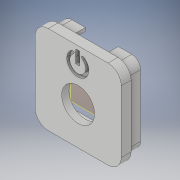
# Autodesk Inventor part: cap
Saved by Autodesk Inventor 2019 (Build 230136000, 136)
## iProperties
Created: 2019-08-20
Part Number: cap
Material: Generic
Document SubType Name: Modeling
Designer: assman
Density: 1 g/cm^3
Appearance: Default
Author: assman
## iProperties of the stored document cap_3DPrint.ipt
Created: 2019-08-20
Part Number: cap_3DPrint
Material: Generic
Document SubType Name: Modeling
Designer: assman
Density: 1 g/cm^3
Appearance: Default
Author: assman
Autodesk Inventor part; units mm, degrees
ref_plane "YZ Plane" through (0, 0, 0) normal (1, 0, 0) x (0, 1, 0)
ref_plane "XZ Plane" through (0, 0, 0) normal (0, 1, 0) x (-1, 0, 0)
ref_plane "XY Plane" through (0, 0, 0) normal (0, 0, 1) x (1, 0, 0)
ref_plane "Work Plane1" through (0, 0, 0) normal (0, 0, 1) x (1, 0, 0)
sketch "Sketch1" plane through (0, 0, 0) normal (0, 0, 1) x (1, 0, 0)
  line L0 (13.075, 9.425) -> (13.075, -9.425) projected
  arc A0 (13.075, 9.425) -> (9.075, 13.425) centre (9.075, 9.425) ccw projected
  line L1 (5, 13.425) -> (9.075, 13.425) projected
  line L2 (-4, 13.425) -> (4, 13.425) projected
  line L3 (5, 13.425) -> (4, 13.425) projected
  line L4 (-4, 13.425) -> (-5, 13.425) projected
  line L5 (-9.075, 13.425) -> (-5, 13.425) projected
  arc A1 (-9.075, 13.425) -> (-13.075, 9.425) centre (-9.075, 9.425) ccw projected
  line L6 (-13.075, -9.425) -> (-13.075, 9.425) projected
  arc A2 (-13.075, -9.425) -> (-9.075, -13.425) centre (-9.075, -9.425) ccw projected
  line L7 (9.075, -13.425) -> (-9.075, -13.425) projected
  arc A3 (9.075, -13.425) -> (13.075, -9.425) centre (9.075, -9.425) ccw projected
  point P0 (0, 0)
extrude "Extrusion1" add sketch "Sketch1" along normal blind 1.2
sketch "Sketch2" plane through (0, 0, 1.2) normal (0, 0, 1) x (1, 0, 0)
  circle A0 centre (0, -2) radius 3.85
  line L0 (-9.075, -13.425) -> (9.075, -13.425)
  point P0 (0, 0)
  dimension "d10" = 13.425
  dimension "d11" = 2
  constraints: 2 end point, 1 centre point
  measures "d10" distance from line of L0 point (0, 0)
  measures "d11" distance of point (0, 0) A0.centre
extrude "Extrusion2" cut sketch "Sketch2" against normal blind 1.2
sketch "Sketch3" plane through (0, 0, 0) normal (0, 0, -1) x (-1, 0, 0)
  arc A0 (-9.075, 12.225) -> (-11.875, 9.425) centre (-9.075, 9.425) ccw projected
  line L0 (-9.075, 12.225) -> (-5, 12.225) projected
  line L1 (-11.875, -9.425) -> (-11.875, 9.425) projected
  arc A1 (-11.875, -9.425) -> (-9.075, -12.225) centre (-9.075, -9.425) ccw projected
  line L2 (9.075, -12.225) -> (-9.075, -12.225) projected
  arc A2 (9.075, -12.225) -> (11.875, -9.425) centre (9.075, -9.425) ccw projected
  line L3 (11.875, 9.425) -> (11.875, -9.425) projected
  arc A3 (11.875, 9.425) -> (9.075, 12.225) centre (9.075, 9.425) ccw projected
  line L4 (5, 12.225) -> (9.075, 12.225) projected
  line L5 (5, 12.125) -> (9.075, 12.125)
  arc A4 (11.775, 9.425) -> (9.075, 12.125) centre (9.075, 9.425) ccw
  line L6 (11.775, 9.425) -> (11.775, -9.425)
  arc A5 (9.075, -12.125) -> (11.775, -9.425) centre (9.075, -9.425) ccw
  line L7 (9.075, -12.125) -> (-9.075, -12.125)
  arc A6 (-11.775, -9.425) -> (-9.075, -12.125) centre (-9.075, -9.425) ccw
  line L8 (-11.775, -9.425) -> (-11.775, 9.425)
  arc A7 (-9.075, 12.125) -> (-11.775, 9.425) centre (-9.075, 9.425) ccw
  line L9 (-9.075, 12.125) -> (-5, 12.125)
  line L10 (5, 11.125) -> (9.075, 11.125)
  arc A8 (10.775, 9.425) -> (9.075, 11.125) centre (9.075, 9.425) ccw
  line L11 (10.775, 9.425) -> (10.775, -9.425)
  arc A9 (9.075, -11.125) -> (10.775, -9.425) centre (9.075, -9.425) ccw
  line L12 (9.075, -11.125) -> (-9.075, -11.125)
  arc A10 (-10.775, -9.425) -> (-9.075, -11.125) centre (-9.075, -9.425) ccw
  line L13 (-10.775, -9.425) -> (-10.775, 9.425)
  arc A11 (-9.075, 11.125) -> (-10.775, 9.425) centre (-9.075, 9.425) ccw
  line L14 (-9.075, 11.125) -> (-5, 11.125)
  line L15 (-5, 12.125) -> (-5, 11.125)
  line L16 (5, 12.125) -> (5, 11.125)
  point P0 (0, 0)
  dimension "d5" = 0.1
  dimension "d6" = 1
  constraints: 24 end point, 16 point on circle, 8 centre point, 1 parallel, 1 vertical, 16 other
  measures "d5" radial gap between concentric circles of A0 A7
  measures "d6" radial gap between concentric circles of A7 A11
extrude "Extrusion3" add sketch "Sketch3" along normal blind 5
sketch "Sketch4" plane through (0, 0, 1.2) normal (0, 0, 1) x (1, 0, 0)
  circle A0 centre (0, -2) radius 3.85 construction
  circle A1 centre (0, -2) radius 5
  point P0 (0, 0)
  dimension "d12" = 10
  constraints: 1 centre point, 1 coincident
  measures "d12" diameter of A1
extrude "Extrusion4" cut sketch "Sketch4" against normal blind 10
sketch "Sketch5" plane through (0, 0, 1.2) normal (0, 0, 1) x (1, 0, 0)
  circle A0 centre (0, -2) radius 5 projected
  line L0 (13.075, -9.425) -> (13.075, 9.425) projected
  arc A1 (13.075, 9.425) -> (9.075, 13.425) centre (9.075, 9.425) ccw projected
  line L1 (9.075, 13.425) -> (-9.075, 13.425) projected
  arc A2 (-9.075, 13.425) -> (-13.075, 9.425) centre (-9.075, 9.425) ccw projected
  line L2 (-13.075, 9.425) -> (-13.075, -9.425) projected
  arc A3 (-13.075, -9.425) -> (-9.075, -13.425) centre (-9.075, -9.425) ccw projected
  line L3 (-9.075, -13.425) -> (9.075, -13.425) projected
  arc A4 (9.075, -13.425) -> (13.075, -9.425) centre (9.075, -9.425) ccw projected
  point P0 (0, 0)
extrude "Extrusion5" add sketch "Sketch5" along normal blind 1
sketch "Sketch6" plane through (0, 0, 0) normal (0, 0, -1) x (-1, 0, 0)
  arc A0 (-9.075, 13.425) -> (-13.075, 9.425) centre (-9.075, 9.425) ccw projected
  line L0 (-13.075, 9.425) -> (-13.075, -9.425) projected
  arc A1 (-13.075, -9.425) -> (-9.075, -13.425) centre (-9.075, -9.425) ccw projected
  line L1 (-9.075, -13.425) -> (9.075, -13.425) projected
  arc A2 (9.075, -13.425) -> (13.075, -9.425) centre (9.075, -9.425) ccw projected
  line L2 (13.075, -9.425) -> (13.075, 9.425) projected
  arc A3 (13.075, 9.425) -> (9.075, 13.425) centre (9.075, 9.425) ccw projected
  line L3 (9.075, 13.425) -> (-9.075, 13.425) projected
  line L4 (-5, 12.125) -> (-9.075, 12.125) projected
  arc A4 (-9.075, 12.125) -> (-11.775, 9.425) centre (-9.075, 9.425) ccw projected
  line L5 (-11.775, 9.425) -> (-11.775, -9.425) projected
  arc A5 (-11.775, -9.425) -> (-9.075, -12.125) centre (-9.075, -9.425) ccw projected
  line L6 (-9.075, -12.125) -> (9.075, -12.125) projected
  arc A6 (9.075, -12.125) -> (11.775, -9.425) centre (9.075, -9.425) ccw projected
  line L7 (11.775, -9.425) -> (11.775, 9.425) projected
  arc A7 (11.775, 9.425) -> (9.075, 12.125) centre (9.075, 9.425) ccw projected
  line L8 (9.075, 12.125) -> (5, 12.125) projected
  line L9 (-5, 12.125) -> (5, 12.125)
  point P0 (0, 0)
  constraints: 2 end point, 1 horizontal
extrude "Extrusion6" add sketch "Sketch6" along normal blind 0.8
sketch "Sketch7" plane through (0, 0, 2.2) normal (0, 0, 1) x (1, 0, 0)
  line L0 (-4.3978, 12.3352) -> (4.3978, 12.3352) construction
  line L1 (4.3978, 12.3352) -> (4.3978, 5.3989) construction
  line L2 (4.3978, 5.3989) -> (-4.3978, 5.3989) construction
  line L3 (-4.3978, 5.3989) -> (-4.3978, 12.3352) construction
  line L4 (0, -18.795) -> (0, 18.795) projected
  spline S0 degree 2 poles (-2.3788, 10.9588) (-1.9786, 11.3515) (-1.3128, 11.4189) (-1.2418, 11.086) knots 0 0 0 1 2 2 2
  spline S1 degree 2 poles (-1.2418, 11.086) (-1.1857, 10.798) (-1.657, 10.3753) knots 0 0 0 1 1 1
  spline S2 degree 2 poles (-1.657, 10.3753) (-2.3452, 9.7432) (-2.6444, 8.1947) (-2.2292, 7.4055) knots 0 0 0 1 2 2 2
  spline S3 degree 2 poles (-2.2292, 7.4055) (-1.93, 6.8557) (-0.6807, 6.0627) (0.475, 6.0627) (1.728, 6.8557) (2.0123, 7.4055) knots 0 0 0 1 2 3 4 4 4
  spline S4 degree 2 poles (2.0123, 7.4055) (2.4387, 8.1947) (2.1507, 9.732) (1.4625, 10.3641) knots 0 0 0 1 2 2 2
  spline S5 degree 2 poles (1.4625, 10.3641) (1.0735, 10.7194) (1.0286, 11.3403) (1.4064, 11.3964) knots 0 0 0 1 2 2 2
  spline S6 degree 2 poles (1.4064, 11.3964) (1.657, 11.4301) (2.6444, 10.5474) (2.895, 10.0424) knots 0 0 0 1 2 2 2
  spline S7 degree 2 poles (2.895, 10.0424) (3.355, 9.1597) (3.0222, 6.9342) (2.3115, 6.2124) knots 0 0 0 1 2 2 2
  spline S8 degree 2 poles (2.3115, 6.2124) (1.7841, 5.6625) (0.4301, 5.1464) (-0.8752, 5.2137) (-2.1133, 5.7785) (-3.0109, 6.7061) (-3.4897, 8.0488) (-3.4112, 8.8044) knots 0 0 0 1 2 3 4 5 6 6 6
  spline S9 degree 2 poles (-3.4112, 8.8044) (-3.3289, 9.515) (-2.8838, 10.4688) (-2.3788, 10.9588) knots 0 0 0 1 2 2 2
  spline S10 degree 2 poles (-0.7518, 10.1584) (-0.7855, 11.935) (-0.6246, 12.3352) (-0.0636, 12.2903) knots 0 0 0 1 2 2 2
  line L5 (-0.0636, 12.2903) -> (0.49, 12.2455)
  line L6 (0.49, 12.2455) -> (0.49, 10.308)
  line L7 (0.49, 10.308) -> (0.49, 8.3668)
  line L8 (0.49, 8.3668) -> (-0.1085, 8.3668)
  line L9 (-0.1085, 8.3668) -> (-0.7032, 8.3668)
  line L10 (-0.7032, 8.3668) -> (-0.7518, 10.1584)
  point P0 (0, 0)
  point P1 (0, 12.3352)
  constraints: 1 midpoint, 1 point on line, 2 other
extrude "Extrusion7" cut sketch "Sketch7" against normal blind 1
body "Solid1"
